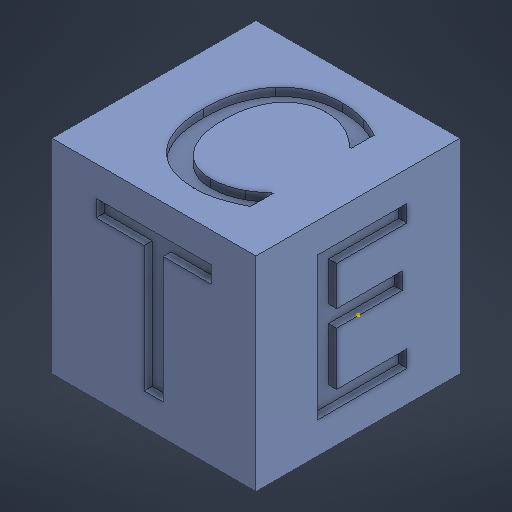
# Autodesk Inventor part: Cubo
Saved by Autodesk Inventor 2025.2 (Build 292293000, 293)
## iProperties
Created: 2025-01-18
Part Number: Cubo
Material: Rubber
Document SubType Name: Modeling
Designer: kenne
Density: 0.93 g/cm^3
Appearance: Rubber - Blue
Author: kenne
Autodesk Inventor part; units mm, degrees
ref_plane "YZ Plane" through (0, 0, 0) normal (1, 0, 0) x (0, 1, 0)
ref_plane "XZ Plane" through (0, 0, 0) normal (0, 1, 0) x (-1, 0, 0)
ref_plane "XY Plane" through (0, 0, 0) normal (0, 0, 1) x (1, 0, 0)
sketch "Sketch1" plane through (0, 0, 0) normal (1, 0, 0) x (0, 1, 0)
  line L0 (12.7, 12.7) -> (-12.7, 12.7)
  line L1 (-12.7, 12.7) -> (-12.7, -12.7)
  line L2 (-12.7, -12.7) -> (12.7, -12.7)
  line L3 (12.7, -12.7) -> (12.7, 12.7)
  line L4 (12.7, 12.7) -> (-12.7, -12.7) construction
  line L5 (-12.7, 12.7) -> (12.7, -12.7) construction
  point P0 (0, 0)
  dimension "d0" = 25.4
  constraints: 12 end point, 2 midpoint, 2 parallel, 2 perpendicular, 1 horizontal
  measures "d0" distance of L2.end L0.start
extrude "Extrusion1" add sketch "Sketch1" along normal mid plane 25.4
sketch "Sketch2" plane through (-12.7, -12.7, 12.7) normal (0, 0, 1) x (1, 0, 0)
  line L0 (5.5252, 21.6747) -> (19.8183, 21.6747) construction
  line L1 (19.8183, 21.6747) -> (19.8183, 3.8947) construction
  line L2 (19.8183, 3.8947) -> (5.5252, 3.8947) construction
  line L3 (5.5252, 3.8947) -> (5.5252, 21.6747) construction
  line L4 (11.4759, 3.8947) -> (11.4759, 19.5711)
  line L5 (11.4759, 19.5711) -> (5.5108, 19.5711)
  line L6 (5.5108, 19.5711) -> (5.5108, 21.6747)
  line L7 (5.5108, 21.6747) -> (19.8039, 21.6747)
  line L8 (19.8039, 21.6747) -> (19.8039, 19.5711)
  line L9 (19.8039, 19.5711) -> (13.8388, 19.5711)
  line L10 (13.8388, 19.5711) -> (13.8388, 3.8947)
  line L11 (13.8388, 3.8947) -> (11.4759, 3.8947)
  point P0 (12.7, 12.7)
  constraints: 2 other
extrude "Extrusion2" cut sketch "Sketch2" against normal blind 1
sketch "Sketch3" plane through (12.7, 0, 0) normal (1, 0, 0) x (0, 0, -1)
  point P0 (0, 0)
sketch "Sketch4" plane through (12.7, 0, 0) normal (1, 0, 0) x (0, 0, -1)
  line L0 (-6.8302, 8.9747) -> (6.8866, 8.9747) construction
  line L1 (6.8866, 8.9747) -> (6.8866, -8.8053) construction
  line L2 (6.8866, -8.8053) -> (-6.8302, -8.8053) construction
  line L3 (-6.8302, -8.8053) -> (-6.8302, 8.9747) construction
  line L4 (-5.0291, -8.8053) -> (-5.0291, 8.9747)
  line L5 (-5.0291, 8.9747) -> (6.0942, 8.9747)
  line L6 (6.0942, 8.9747) -> (6.0942, 6.8711)
  line L7 (6.0942, 6.8711) -> (-2.6661, 6.8711)
  line L8 (-2.6661, 6.8711) -> (-2.6661, 2.001)
  line L9 (-2.6661, 2.001) -> (5.5034, 2.001)
  line L10 (5.5034, 2.001) -> (5.5034, -0.1026)
  line L11 (5.5034, -0.1026) -> (-2.6661, -0.1026)
  line L12 (-2.6661, -0.1026) -> (-2.6661, -6.7017)
  line L13 (-2.6661, -6.7017) -> (6.0942, -6.7017)
  line L14 (6.0942, -6.7017) -> (6.0942, -8.8053)
  line L15 (6.0942, -8.8053) -> (-5.0291, -8.8053)
  point P0 (0, 0)
  constraints: 2 other
extrude "Extrusion3" cut sketch "Sketch4" against normal blind 1
sketch "Sketch5" plane through (12.7, 12.7, -12.7) normal (0, 0, -1) x (-1, 0, 0)
  line L0 (5.2226, -3.6687) -> (20.1209, -3.6687) construction
  line L1 (20.1209, -3.6687) -> (20.1209, -21.4487) construction
  line L2 (20.1209, -21.4487) -> (5.2226, -21.4487) construction
  line L3 (5.2226, -21.4487) -> (5.2226, -3.6687) construction
  line L4 (5.1073, -21.4487) -> (11.1012, -3.6687)
  line L5 (11.1012, -3.6687) -> (14.0117, -3.6687)
  line L6 (14.0117, -3.6687) -> (20.0056, -21.4487)
  line L7 (20.0056, -21.4487) -> (17.513, -21.4487)
  line L8 (17.513, -21.4487) -> (15.8992, -16.4778)
  line L9 (15.8992, -16.4778) -> (9.1129, -16.4778)
  line L10 (9.1129, -16.4778) -> (7.4991, -21.4487)
  line L11 (7.4991, -21.4487) -> (5.1073, -21.4487)
  line L12 (15.2508, -14.4606) -> (12.4988, -6.0893)
  line L13 (12.4988, -6.0893) -> (9.7612, -14.4606)
  line L14 (9.7612, -14.4606) -> (15.2508, -14.4606)
  point P0 (12.7, -12.7)
  constraints: 2 other
extrude "Extrusion4" cut sketch "Sketch5" against normal blind 1
sketch "Sketch6" plane through (-12.7, 0, 0) normal (-1, 0, 0) x (0, 0, 1)
  line L0 (-7.6143, 8.9183) -> (7.5578, 8.9183) construction
  line L1 (7.5578, 8.9183) -> (7.5578, -8.8617) construction
  line L2 (7.5578, -8.8617) -> (-7.6143, -8.8617) construction
  line L3 (-7.6143, -8.8617) -> (-7.6143, 8.9183) construction
  line L4 (7.9468, -8.8617) -> (4.8778, -8.8617)
  line L5 (4.8778, -8.8617) -> (-0.7415, -1.7872)
  line L6 (-0.7415, -1.7872) -> (-3.4503, -1.7872)
  line L7 (-3.4503, -1.7872) -> (-3.4503, -8.8617)
  line L8 (-3.4503, -8.8617) -> (-5.8132, -8.8617)
  line L9 (-5.8132, -8.8617) -> (-5.8132, 8.9183)
  line L10 (-5.8132, 8.9183) -> (-1.2314, 8.9183)
  spline S0 degree 2 poles (-1.2314, 8.9183) (0.2959, 8.9183) (2.3563, 8.5869) (3.2929, 7.9817) knots 0 0 0 1 2 2 2
  spline S1 degree 2 poles (3.2929, 7.9817) (4.2294, 7.3766) (5.3101, 5.4891) (5.3101, 4.0914) knots 0 0 0 1 2 2 2
  spline S2 degree 2 poles (5.3101, 4.0914) (5.3101, 2.1463) (3.3217, -0.4904) (1.6215, -1.1244) knots 0 0 0 1 2 2 2
  line L11 (1.6215, -1.1244) -> (7.9468, -8.8617)
  spline S3 degree 2 poles (2.8462, 3.9041) (2.8462, 4.6822) (2.2987, 5.8781) (1.7224, 6.2671) knots 0 0 0 1 2 2 2
  spline S4 degree 2 poles (1.7224, 6.2671) (1.2181, 6.5985) (-0.1219, 6.8723) (-1.1017, 6.8723) knots 0 0 0 1 2 2 2
  line L12 (-1.1017, 6.8723) -> (-3.4503, 6.8723)
  line L13 (-3.4503, 6.8723) -> (-3.4503, 0.1868)
  line L14 (-3.4503, 0.1868) -> (-1.3754, 0.1868)
  spline S5 degree 2 poles (-1.3754, 0.1868) (-0.3524, 0.1868) (1.2757, 0.547) (1.8376, 1.1089) knots 0 0 0 1 2 2 2
  spline S6 degree 2 poles (1.8376, 1.1089) (2.3563, 1.5988) (2.8462, 2.982) (2.8462, 3.9041) knots 0 0 0 1 2 2 2
  point P0 (0, 0)
  constraints: 2 other
extrude "Extrusion5" cut sketch "Sketch6" against normal blind 1
sketch "Sketch7" plane through (-12.7, 12.7, 12.7) normal (0, 1, 0) x (1, 0, 0)
  line L0 (5.4437, 21.8787) -> (20.1259, 21.8787) construction
  line L1 (20.1259, 21.8787) -> (20.1259, 3.4648) construction
  line L2 (20.1259, 3.4648) -> (5.4437, 3.4648) construction
  line L3 (5.4437, 3.4648) -> (5.4437, 21.8787) construction
  spline S0 degree 2 poles (14.1896, 3.4648) (12.4606, 3.4648) (9.5357, 4.6318) (8.4695, 5.7989) knots 0 0 0 1 2 2 2
  spline S1 degree 2 poles (8.4695, 5.7989) (7.4032, 6.9516) (6.2361, 10.4096) (6.2361, 12.6573) knots 0 0 0 1 2 2 2
  spline S2 degree 2 poles (6.2361, 12.6573) (6.2361, 14.8906) (7.3744, 18.2046) (8.455, 19.4293) knots 0 0 0 1 2 2 2
  spline S3 degree 2 poles (8.455, 19.4293) (9.5213, 20.6252) (12.4318, 21.8787) (14.2328, 21.8787) knots 0 0 0 1 2 2 2
  spline S4 degree 2 poles (14.2328, 21.8787) (15.1261, 21.8787) (16.6967, 21.6194) (17.3595, 21.4177) knots 0 0 0 1 2 2 2
  spline S5 degree 2 poles (17.3595, 21.4177) (17.9358, 21.2303) (19.1317, 20.6972) (19.7224, 20.3802) knots 0 0 0 1 2 2 2
  line L4 (19.7224, 20.3802) -> (19.7224, 17.5274)
  line L5 (19.7224, 17.5274) -> (19.5351, 17.5274)
  spline S6 degree 2 poles (19.5351, 17.5274) (19.2181, 17.8155) (18.2384, 18.6224) (17.5324, 19.0114) knots 0 0 0 1 2 2 2
  spline S7 degree 2 poles (17.5324, 19.0114) (16.8552, 19.3861) (15.2558, 19.8615) (14.2184, 19.8615) knots 0 0 0 1 2 2 2
  spline S8 degree 2 poles (14.2184, 19.8615) (13.0802, 19.8615) (11.0486, 18.925) (10.2849, 18.0317) knots 0 0 0 1 2 2 2
  spline S9 degree 2 poles (10.2849, 18.0317) (9.5357, 17.1239) (8.7, 14.3719) (8.7, 12.6573) knots 0 0 0 1 2 2 2
  spline S10 degree 2 poles (8.7, 12.6573) (8.7, 10.8275) (9.5789, 8.1907) (10.3426, 7.283) knots 0 0 0 1 2 2 2
  spline S11 degree 2 poles (10.3426, 7.283) (11.0918, 6.4041) (13.0946, 5.5108) (14.2184, 5.5108) knots 0 0 0 1 2 2 2
  spline S12 degree 2 poles (14.2184, 5.5108) (15.2414, 5.5108) (16.9848, 6.015) (17.662, 6.3897) knots 0 0 0 1 2 2 2
  spline S13 degree 2 poles (17.662, 6.3897) (18.3104, 6.7643) (19.2758, 7.5423) (19.5495, 7.8161) knots 0 0 0 1 2 2 2
  line L6 (19.5495, 7.8161) -> (19.7224, 7.8161)
  line L7 (19.7224, 7.8161) -> (19.7224, 4.992)
  spline S14 degree 2 poles (19.7224, 4.992) (19.1317, 4.7183) (18.0943, 4.214) (17.3595, 3.9835) knots 0 0 0 1 2 2 2
  spline S15 degree 2 poles (17.3595, 3.9835) (16.5814, 3.7241) (15.2558, 3.4648) (14.1896, 3.4648) knots 0 0 0 1 2 2 2
  point P0 (12.7, 12.7)
  constraints: 2 other
extrude "Extrusion6" cut sketch "Sketch7" against normal blind 1
sketch "Sketch8" plane through (-12.7, -12.7, -12.7) normal (0, -1, 0) x (1, 0, 0)
  line L0 (8.055, 21.6183) -> (17.1755, 21.6183) construction
  line L1 (17.1755, 21.6183) -> (17.1755, 3.8383) construction
  line L2 (17.1755, 3.8383) -> (8.055, 3.8383) construction
  line L3 (8.055, 3.8383) -> (8.055, 21.6183) construction
  line L4 (16.0516, 3.8383) -> (9.1644, 3.8383)
  line L5 (9.1644, 3.8383) -> (9.1644, 5.6537)
  line L6 (9.1644, 5.6537) -> (11.4265, 5.6537)
  line L7 (11.4265, 5.6537) -> (11.4265, 19.8028)
  line L8 (11.4265, 19.8028) -> (9.1644, 19.8028)
  line L9 (9.1644, 19.8028) -> (9.1644, 21.6183)
  line L10 (9.1644, 21.6183) -> (16.0516, 21.6183)
  line L11 (16.0516, 21.6183) -> (16.0516, 19.8028)
  line L12 (16.0516, 19.8028) -> (13.7895, 19.8028)
  line L13 (13.7895, 19.8028) -> (13.7895, 5.6537)
  line L14 (13.7895, 5.6537) -> (16.0516, 5.6537)
  line L15 (16.0516, 5.6537) -> (16.0516, 3.8383)
  point P0 (12.7, 12.7)
  constraints: 2 other
extrude "Extrusion7" cut sketch "Sketch8" against normal blind 1
equation "\"d1\" = d0"
